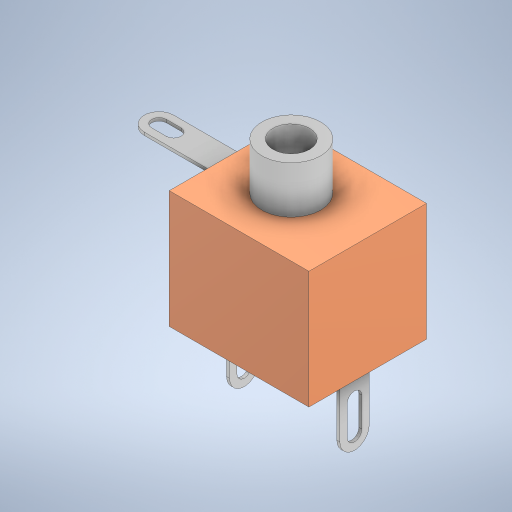
# Autodesk Inventor part: 2.5mm jack
Saved by Autodesk Inventor 2024 (Build 280153000, 153)
## iProperties
Created: 2025-09-12
Part Number: 2.5mm jack
Material: Generic
Document SubType Name: Modeling
Designer: Login
Density: 1 g/cm^3
Appearance: Default
Author: Login
Autodesk Inventor part; units mm, degrees
ref_plane "YZ Plane" through (0, 0, 0) normal (1, 0, 0) x (0, 1, 0)
ref_plane "XZ Plane" through (0, 0, 0) normal (0, 1, 0) x (-1, 0, 0)
ref_plane "XY Plane" through (0, 0, 0) normal (0, 0, 1) x (1, 0, 0)
sketch "Sketch1" plane through (0, 0, 0) normal (0, 1, 0) x (-1, 0, 0)
  line L0 (4.75, 4) -> (-4.75, 4)
  line L1 (-4.75, 4) -> (-4.75, -4)
  line L2 (-4.75, -4) -> (4.75, -4)
  line L3 (4.75, -4) -> (4.75, 4)
  line L4 (4.75, 4) -> (-4.75, -4) construction
  line L5 (-4.75, 4) -> (4.75, -4) construction
  point P0 (0, 0)
  dimension "d0" = 9.5
  dimension "d1" = 8
  constraints: 12 end point, 2 midpoint, 2 parallel, 1 horizontal, 1 perpendicular
  measures "d0" distance of L2.end L1.end
  measures "d1" distance of L1.end L0.end
extrude "Extrusion1" add sketch "Sketch1" along normal blind 8
sketch "Sketch2" plane through (0, 8, 0) normal (0, 1, 0) x (1, 0, 0)
  circle A0 centre (-0.45, 0) radius 2
  line L0 (-4.75, 4) -> (-4.75, -4) projected
  line L1 (4.75, 4) -> (-4.75, 4) projected
  point P0 (0, 0)
  dimension "d4" = 4
  dimension "d5" = 4.3
  dimension "d6" = 4
  constraints: 1 centre point
  measures "d4" diameter of A0
  measures "d5" distance from line of L0 A0.centre
  measures "d6" distance from line of L1 A0.centre
extrude "Extrusion2" add sketch "Sketch2" along normal blind 3.2
sketch "Sketch3" plane through (-0.45, 11.2, 0) normal (0, 1, 0) x (1, 0, 0)
  point P0 (0.45, 0)
  point P1 (0, 0)
hole "Hole1" at (-0.45, 11.2, 0) direction (0, -1, 0) diameter 2.5 depth 8
sketch "Sketch4" plane through (0, 0, 0) normal (0, -1, 0) x (1, 0, 0)
  line L0 (-3.65, -1) -> (-3.85, -1)
  line L1 (-3.85, -1) -> (-3.85, 1)
  line L2 (-3.85, 1) -> (-3.65, 1)
  line L3 (-3.65, 1) -> (-3.65, -1)
  line L4 (-3.65, -1) -> (-3.85, 1) construction
  line L5 (-3.85, -1) -> (-3.65, 1) construction
  line L6 (3.65, -1) -> (3.85, -1)
  line L7 (3.85, -1) -> (3.85, 1)
  line L8 (3.85, 1) -> (3.65, 1)
  line L9 (3.65, 1) -> (3.65, -1)
  line L10 (3.65, -1) -> (3.85, 1) construction
  line L11 (3.85, -1) -> (3.65, 1) construction
  line L12 (4.75, 4) -> (4.75, -4) projected
  line L13 (-4.75, 4) -> (4.75, 4) projected
  point P0 (0, 0)
  point P1 (-3.75, 0)
  point P2 (3.75, 0)
  point P3 (3.65, 0)
  dimension "d16" = 0.2
  dimension "d17" = 2
  dimension "d18" = 0.2
  dimension "d19" = 2
  dimension "d20" = 7.5
  dimension "d21" = 1
  dimension "d22" = 4
  constraints: 24 end point, 5 midpoint, 4 parallel, 2 horizontal, 2 perpendicular, 1 collinear
  measures "d16" distance of L1.end L2.end
  measures "d17" distance of L0.end L1.end
  measures "d18" distance of L8.end L7.end
  measures "d19" distance of L7.end L6.end
  measures "d20" distance of point (-3.75, 0) point (3.75, 0)
  measures "d21" distance from line of L12 point (3.75, 0)
  measures "d22" distance from line of L13 point (3.65, 0)
extrude "Extrusion3" add sketch "Sketch4" along normal blind 5
fillet "Fillet1" radius 1 4 edges at (3.75, -5, -1) (3.75, -5, 1) (-3.75, -5, 1) (-3.75, -5, -1)
sketch "Sketch5" plane through (3.85, 0, 1) normal (1, 0, 0) x (0, 0, -1)
  line L0 (1, -2) -> (1, -4) construction
  line L1 (1.5, -2) -> (1.5, -4)
  line L2 (0.5, -4) -> (0.5, -2)
  arc A0 (1.5, -2) -> (0.5, -2) centre (1, -2) ccw
  arc A1 (0.5, -4) -> (1.5, -4) centre (1, -4) ccw
  line L3 (0, 0) -> (0, -4) projected
  arc A2 (0, -4) -> (2, -4) centre (1, -4) ccw projected
  point P0 (1, 0)
  point P1 (1, -3)
  dimension "d26" = 1
  dimension "d27" = 1
  dimension "d28" = 0.5
  dimension "d29" = 0.5
  constraints: 8 end point, 4 point on circle, 4 tangent, 2 centre point, 1 midpoint, 1 parallel, 1 vertical
  measures "d26" distance of point (1, -3) L0.end
  measures "d27" distance between parallel lines of L1 L2
  measures "d28" distance between parallel lines of L3 L2
  measures "d29" radial gap between concentric circles of A2 A1
extrude "Extrusion4" cut sketch "Sketch5" against normal through all
sketch "Sketch6" plane through (-4.75, 0, -4) normal (-1, 0, 0) x (0, 0, 1)
  line L0 (3, 7.6) -> (5, 7.6)
  line L1 (5, 7.6) -> (5, 7.4)
  line L2 (5, 7.4) -> (3, 7.4)
  line L3 (3, 7.4) -> (3, 7.6)
  line L4 (3, 7.6) -> (5, 7.4) construction
  line L5 (5, 7.6) -> (3, 7.4) construction
  line L6 (0, 0) -> (0, 8) projected
  line L7 (0, 8) -> (8, 8) projected
  point P0 (4, 0)
  point P1 (4, 7.5)
  dimension "d32" = 2
  dimension "d33" = 0.2
  dimension "d34" = 4
  dimension "d35" = 0.5
  constraints: 12 end point, 2 midpoint, 2 parallel, 1 horizontal, 1 perpendicular
  measures "d32" distance of L1.end L2.end
  measures "d33" distance of L0.end L1.end
  measures "d34" distance from line of L6 point (4, 7.5)
  measures "d35" distance from line of L7 point (4, 7.5)
extrude "Extrusion5" add sketch "Sketch6" along normal blind 5.7
fillet "Fillet2" radius 1 2 edges at (-10.45, 7.5, 1) (-10.45, 7.5, -1)
sketch "Sketch7" plane through (-4.75, 7.6, 1) normal (0, 1, 0) x (1, 0, 0)
  line L0 (-4.7, 1) -> (-3.7, 1) construction
  line L1 (-4.7, 0.5) -> (-3.7, 0.5)
  line L2 (-3.7, 1.5) -> (-4.7, 1.5)
  arc A0 (-4.7, 1.5) -> (-4.7, 0.5) centre (-4.7, 1) ccw
  arc A1 (-3.7, 0.5) -> (-3.7, 1.5) centre (-3.7, 1) ccw
  line L3 (0, 2) -> (-4.7, 2) projected
  arc A2 (-4.7, 2) -> (-4.7, 0) centre (-4.7, 1) ccw projected
  point P0 (4.75, 1)
  point P1 (-4.2, 1)
  dimension "d39" = 0.5
  dimension "d40" = 1
  dimension "d41" = 0.5
  dimension "d42" = 0.5
  constraints: 8 end point, 4 point on circle, 4 tangent, 2 centre point, 1 horizontal, 1 midpoint, 1 parallel
  measures "d39" distance of point (-4.2, 1) L0.end
  measures "d40" diameter of A1
  measures "d41" distance between parallel lines of L3 L2
  measures "d42" radial gap between concentric circles of A2 A0
extrude "Extrusion6" cut sketch "Sketch7" against normal through all
body "Solid1"
